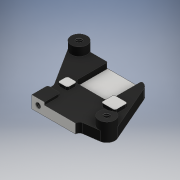
# Autodesk Inventor part: EPS_RegulatorHeatsink-B
Saved by Autodesk Inventor 2018 (Build 220112000, 112)
## iProperties
Created: 2018-09-29
Part Number: EPS_RegulatorHeatsink-B
Material: Aluminum 6061
Document SubType Name: Modeling
Designer: Bradley
Density: 2.7 g/cm^3
Appearance: Anodized - Dark Gray
Mass: 1.86381 g
Surface Area: 8.94347 cm^2
Volume: 0.6903 cm^3
Author: Bradley
Autodesk Inventor part; units mm, degrees
ref_plane "YZ Plane" through (0, 0, 0) normal (1, 0, 0) x (0, 1, 0)
ref_plane "XZ Plane" through (0, 0, 0) normal (0, 1, 0) x (-1, 0, 0)
ref_plane "XY Plane" through (0, 0, 0) normal (0, 0, 1) x (1, 0, 0)
sketch "Sketch7" plane through (0, 0, 0) normal (0, 0, 1) x (1, 0, 0)
  line L0 (-3.75, -3.75) -> (3.75, -3.75) construction
  line L1 (3.75, -3.75) -> (3.75, 3.75) construction
  line L2 (3.75, 3.75) -> (-3.75, 3.75) construction
  line L3 (-3.75, 3.75) -> (-3.75, -3.75) construction
  line L4 (-3.75, -3.75) -> (3.75, 3.75) construction
  line L5 (3.75, -3.75) -> (-3.75, 3.75) construction
  line L6 (7.875, -6.175) -> (4.725, -6.175) construction
  line L7 (4.725, -6.175) -> (4.725, -3.025) construction
  line L8 (4.725, -3.025) -> (7.875, -3.025) construction
  line L9 (7.875, -3.025) -> (7.875, -6.175) construction
  line L10 (7.875, -6.175) -> (4.725, -3.025) construction
  line L11 (4.725, -6.175) -> (7.875, -3.025) construction
  line L12 (-3.275, -4.95) -> (-5.225, -4.95) construction
  line L13 (-5.225, -4.95) -> (-5.225, -6.85) construction
  line L14 (-5.225, -6.85) -> (-3.275, -6.85) construction
  line L15 (-3.275, -6.85) -> (-3.275, -4.95) construction
  line L16 (-3.275, -4.95) -> (-5.225, -6.85) construction
  line L17 (-5.225, -4.95) -> (-3.275, -6.85) construction
  circle A0 centre (9.4, -9.6) radius 2
  circle A1 centre (-10.5, 3.3) radius 2
  line L18 (5.05, -2.975) -> (7.55, -2.975)
  line L19 (8.05, -3.475) -> (8.05, -5.725)
  line L20 (7.55, -6.225) -> (5.05, -6.225)
  line L21 (4.55, -5.725) -> (4.55, -3.475)
  arc A2 (5.05, -2.975) -> (4.55, -3.475) centre (5.05, -3.475) ccw
  arc A3 (4.55, -5.725) -> (5.05, -6.225) centre (5.05, -5.725) ccw
  arc A4 (7.55, -6.225) -> (8.05, -5.725) centre (7.55, -5.725) ccw
  arc A5 (8.05, -3.475) -> (7.55, -2.975) centre (7.55, -3.475) ccw
  line L22 (7.55, -5.725) -> (9.4, -9.6) construction
  circle A6 centre (8.2393, -7.1689) radius 1.1 construction
  line L23 (9.8034, -7.6411) -> (7.6231, -8.682)
  line L24 (-8.74, 4.25) -> (4.25, 4.25)
  arc A7 (6.0843, 3.0472) -> (4.25, 4.25) centre (4.25, 2.25) ccw
  line L25 (6.0843, 3.0472) -> (11.2343, -8.8028)
  line L26 (-12.1884, 2.228) -> (-6.3116, -7.028)
  arc A8 (-6, -8.1) -> (-6.3116, -7.028) centre (-8, -8.1) ccw
  line L27 (-6, -8.1) -> (-6, -13.1)
  line L28 (-6, -13.1) -> (5, -13.1)
  arc A9 (5.8627, -12.1095) -> (5, -13.1) centre (6, -13.1) ccw
  line L29 (5.8627, -12.1095) -> (9.6746, -11.5811)
  line L30 (-4.25, 4.25) -> (-4.25, -3.25)
  arc A10 (-4.25, -3.25) -> (-3.25, -4.25) centre (-3.25, -3.25) ccw
  line L31 (-3.25, -4.25) -> (3.25, -4.25)
  arc A11 (3.25, -4.25) -> (4.25, -3.25) centre (3.25, -3.25) ccw
  line L32 (4.25, -3.25) -> (4.25, 4.25)
  line L33 (-3.5, -7.1179) -> (-5, -7.1179)
  line L34 (-5.5, -6.6179) -> (-5.5, -5.1821)
  line L35 (-5, -4.6821) -> (-3.5, -4.6821)
  line L36 (-3, -5.1821) -> (-3, -6.6179)
  arc A12 (-3.5, -7.1179) -> (-3, -6.6179) centre (-3.5, -6.6179) ccw
  arc A13 (-5.5, -6.6179) -> (-5, -7.1179) centre (-5, -6.6179) ccw
  arc A14 (-5, -4.6821) -> (-5.5, -5.1821) centre (-5, -5.1821) ccw
  arc A15 (-3, -5.1821) -> (-3.5, -4.6821) centre (-3.5, -5.1821) ccw
  line L37 (-2.8, -13.1) -> (-2.8, -9.6)
  arc A16 (-2.8, -9.6) -> (-3.3, -9.1) centre (-3.3, -9.6) ccw
  line L38 (-3.3, -9.1) -> (-5.5, -9.1)
  arc A17 (-5.5, -9.1) -> (-6, -9.6) centre (-5.5, -9.6) ccw
  point P0 (0, 0)
  point P1 (6.3, -4.6)
  point P2 (-4.25, -5.9)
  point P3 (6.3, -2.975)
  point P4 (6.3, -3.025)
  point P5 (4.725, -4.6)
  point P6 (4.55, -4.6)
  point P7 (0, -4.25)
  point P8 (0, 0)
  point P9 (-5.5, -4.6821)
  point P10 (-4.25, -7.1179)
  point P11 (-4.25, -5.9)
  point P12 (-4.25, -5.9)
  point P13 (-3, -5.9)
  dimension "d58" = 7.5
  dimension "d60" = 4.6
  dimension "d61" = 6.3
  dimension "d62" = 3.15
  dimension "d63" = 4.25
  dimension "d64" = 1.95
  dimension "d65" = 1.9
  dimension "d66" = 5.9
  dimension "d67" = 4
  dimension "d68" = 19.9
  dimension "d69" = 12.9
  dimension "d70" = 9.4
  dimension "d71" = 9.6
  dimension "d83" = 0.5
  dimension "d84" = 2.2
  dimension "d85" = 1.594
  dimension "d86" = 3.5
  dimension "d87" = 3.25
  dimension "d88" = 4.25
  dimension "d89" = 2
  dimension "d91" = 13.1
  dimension "d93" = 5
  dimension "d94" = 5
  dimension "d97" = 6
  dimension "d98" = 8.5
  dimension "d99" = 1
  dimension "d100" = 4.25
  dimension "d105" = 0.5
  dimension "d106" = 2.5
  dimension "d109" = 3.2
  dimension "d110" = 4
  constraints: 78 end point, 36 point on circle, 34 tangent, 18 centre point, 16 midpoint, 12 equal radius, 12 parallel, 11 perpendicular, 8 point on line, 6 horizontal, 3 vertical alignment, 2 horizontal alignment, 2 vertical
  measures "d58" distance of L2.end L1.end
  measures "d60" vertical distance of point (6.3, -4.6) point (0, 0)
  measures "d61" horizontal distance of point (0, 0) point (6.3, -4.6)
  measures "d62" distance of L7.end L8.end
  measures "d63" horizontal distance of point (-4.25, -5.9) point (0, 0)
  measures "d64" distance of L13.end L14.end
  measures "d65" distance of L12.end L13.end
  measures "d66" vertical distance of point (-4.25, -5.9) point (0, 0)
  measures "d67" diameter of A0
  measures "d68" horizontal distance of L22.end A1.centre
  measures "d69" vertical distance of L22.end A1.centre
  measures "d70" horizontal distance of L22.end point (0, 0)
  measures "d71" vertical distance of L22.end point (0, 0)
  measures "d83" radius of A2
  measures "d84" diameter of A6
  measures "d85" distance from line of L22.end L23
  measures "d86" distance between parallel lines of L19 L21
  measures "d87" distance between parallel lines of L20 L18
  measures "d88" distance from line of L24 point (0, 0)
  measures "d89" radius of A7
  measures "d91" vertical distance of L27.end point (0, 0)
  measures "d93" horizontal distance of L28.end point (0, 0)
  measures "d94" distance of L27.start L27.end
  measures "d97" distance from line of point (0, 0) L27
  measures "d98" distance between parallel lines of L32 L30
  measures "d99" radius of A10
  measures "d100" distance from line of point (0, 0) L31
  measures "d105" radius of A12
  measures "d106" distance between parallel lines of L34 L36
  measures "d109" distance between parallel lines of L27 L37
  measures "d110" distance between parallel lines of L38 L28
extrude "Extrusion5" add sketch "Sketch7" along normal blind 3.5 and the other way blind 1 contours A0 L23 | A1 picked at (10.0114, -9.3401)
sketch "Sketch8" plane through (-10.5, 3.3, 3.5) normal (0, 0, 1) x (1, 0, 0)
  circle A0 centre (0, 0) radius 2 projected
  arc A1 (18.1231, -11.982) -> (20.3034, -10.9411) centre (19.9, -12.9) ccw projected
  line L0 (20.3034, -10.9411) -> (18.1231, -11.982) projected
  point P0 (10.5, -3.3)
hole "Hole3" at (-10.5, 3.3, 3.5) at (9.4, -9.6, 3.5) direction (0, 0, -1) diameter 1.567 end through all thread size "M2x0.4" class "6H" standard "ANSI Metric M Profile"
extrude "Extrusion6" add sketch "Sketch7" against normal up to surface (1 mm away) contours A0 L29 A9 L28 L37 A16 L38 A17 L27 A8 L26 A1 L24 L30 A10 L31 A11 L32 A7 L25 | L23 A0 | L32 A11 L31 A10 L30 L24 | L28 L27 A17 L38 A16 L37 | L18 A5 L19 A4 L20 A3 L21 A2 | L33 A13 L34 A14 L35 A15 L36 A12 picked at (8.4293, -8.2151)
extrude "Extrusion7" add sketch "Sketch7" along normal blind 1.4 contours A0 L29 A9 L28 L37 A16 L38 A17 L27 A8 L26 A1 L24 L30 A10 L31 A11 L32 A7 L25 | L23 A0 | L28 L27 A17 L38 A16 L37 | L18 A5 L19 A4 L20 A3 L21 A2 | L33 A13 L34 A14 L35 A15 L36 A12 picked at (8.4293, -8.2151)
extrude "Extrusion8" add sketch "Sketch7" along normal blind 2.27 contours L18 A5 L19 A4 L20 A3 L21 A2
extrude "Extrusion9" add sketch "Sketch7" along normal blind 2.15 contours L33 A13 L34 A14 L35 A15 L36 A12
extrude "Extrusion10" add sketch "Sketch7" along normal blind 2.1 contours L28 L27 A17 L38 A16 L37
sketch "Sketch9" plane through (-6, -13.1, -1) normal (0, -1, 0) x (1, 0, 0)
  line L0 (0, 0) -> (0, 3.1) projected
  line L1 (11, 0) -> (0, 0) projected
  line L2 (11, 0) -> (11, 2.4) projected
  line L3 (3.2, 2.4) -> (11, 2.4) projected
  line L4 (3.2, 2.4) -> (3.2, 3.1) projected
  line L5 (0, 3.1) -> (3.2, 3.1) projected
  line L6 (0, 0) -> (3.2, 3.1) construction
  point P0 (6, 1)
  point P1 (1.6, 1.55)
  constraints: 2 end point, 1 midpoint
hole "Hole4" at (-4.4, -13.1, 0.55) direction (0, 1, 0) diameter 1.221 depth 3 tip angle 118 thread size "M1.6x0.35" class "6H" standard "ANSI Metric M Profile"
fillet "Fillet3" radius 0.25 2 edges at (4.25, 4.25, 0.7) (-4.25, 4.25, 0.7)
equation "\"d100\" = 0.5 * d98"
equation "\"SilPad\" = 0.35"
body "Solid2"
